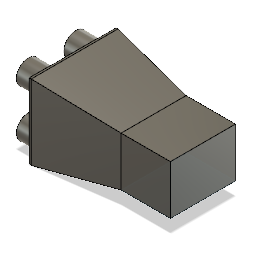
ExtrusionRack_mount_hanging_version (Autodesk Fusion 360 design; units mm, degrees)
Autodesk Fusion 360 part; units mm, degrees
sketch "Sketch1" plane through (0, 0, 0) normal (0, 0, 1) x (1, 0, 0)
  line L0 (10.25, -10.25) -> (-10.25, -10.25)
  line L1 (-10.25, -10.25) -> (-10.25, 10.25)
  line L2 (-10.25, 10.25) -> (10.25, 10.25)
  line L3 (10.25, 10.25) -> (10.25, -10.25)
  line L4 (10.25, -10.25) -> (-10.25, 10.25) construction
  line L5 (-10.25, -10.25) -> (10.25, 10.25) construction
  line L6 (12.5, -12.5) -> (-12.5, -12.5)
  line L7 (-12.5, -12.5) -> (-12.5, 12.5)
  line L8 (-12.5, 12.5) -> (12.5, 12.5)
  line L9 (12.5, 12.5) -> (12.5, -12.5)
  line L10 (12.5, -12.5) -> (-12.5, 12.5) construction
  line L11 (-12.5, -12.5) -> (12.5, 12.5) construction
  dimension "d1" = 20.5
  dimension "d2" = 20.5
  dimension "d3" = 25
  dimension "d4" = 25
  constraint perpendicular L0 L1
  constraint parallel L0 L2
  constraint parallel L1 L3
  constraint horizontal L0
  constraint coincident L4 origin
  constraint coincident L5 origin
  constraint perpendicular L6 L7
  constraint parallel L6 L8
  constraint parallel L7 L9
  constraint horizontal L6
  constraint coincident L10 origin
  constraint coincident L11 origin
  measures "d1" distance of L1.end L2.end
  measures "d2" distance of L0.end L1.end
  measures "d3" distance of L7.end L8.end
  measures "d4" distance of L6.end L7.end
extrude "Extrude1" add sketch "Sketch1" along normal blind 30 makes body 1
sketch "Sketch2" plane through (0, 0, 30) normal (0, 0, 1) x (1, 0, 0)
  line L0 (-10.25, 10.25) -> (10.25, 10.25)
  line L1 (10.25, 10.25) -> (10.25, -10.25)
  line L2 (10.25, -10.25) -> (-10.25, -10.25)
  line L3 (-10.25, -10.25) -> (-10.25, 10.25)
  line L4 (12.5, 12.5) -> (-12.5, 12.5)
  line L5 (-12.5, 12.5) -> (-12.5, -12.5)
  line L6 (-12.5, -12.5) -> (12.5, -12.5)
  line L7 (12.5, -12.5) -> (12.5, 12.5)
  line L8 (-12.5, 12.5) -> (12.5, 12.5)
  line L9 (12.5, 12.5) -> (12.5, -12.5)
  line L10 (12.5, -12.5) -> (-12.5, -12.5)
  line L11 (-12.5, -12.5) -> (-12.5, 12.5)
  constraint horizontal L8
  constraint vertical L9
  constraint horizontal L10
  constraint vertical L11
  constraint coincident L6.end L7.start
  constraint coincident L4.end L5.start
extrude "Extrude2" add sketch "Sketch2" along normal blind 3 contours L0 L1 L2 L3 | L4 L5 L6 L7 L8 L9 L10 L11 bodies 1
sketch "Sketch7" plane through (0, -12.5, 0) normal (0, -1, 0) x (1, 0, 0)
  line L0 (-12.5, 0) -> (12.5, 0)
  line L1 (12.5, 0) -> (12.5, 33)
  line L2 (12.5, 33) -> (-12.5, 33)
  line L3 (-12.5, 33) -> (-12.5, 0)
ref_plane "WorkPlane3" through (0, -0.5, 16.5) normal (0, -1, 0) x (1, 0, 0)
sketch "Sketch8" plane through (0, -0.5, 16.5) normal (0, -1, 0) x (1, 0, 0)
ref_plane "WorkPlane4" through (-52.5, 0, 16.5) normal (-1, 0, 0) x (0, -1, 0)
sketch "Sketch9" plane through (-52.5, 0, 16.5) normal (-1, 0, 0) x (0, 0, -1)
  line L0 (-22, 19) -> (22, 19)
  line L1 (22, 19) -> (22, -19)
  line L2 (22, -19) -> (-22, -19)
  line L3 (-22, -19) -> (-22, 19)
  line L4 (-22, 19) -> (22, -19) construction
  line L5 (22, 19) -> (-22, -19) construction
  constraint perpendicular L0 L1
  constraint parallel L0 L2
  constraint parallel L1 L3
  constraint horizontal L0
  constraint coincident L4 origin
  constraint coincident L5 origin
extrude "Extrude4" add sketch "Sketch9" along normal blind 1 separate body makes body 2
loft "Loft2" add section 1 face at (-12.5, -4.1667, 11) section 2 face at (-52.5, -6.3333, 23.8333) on bodies 1 2 bodies 1 2
sketch "Sketch10" plane through (-53.5, 0, 0) normal (-1, 0, 0) x (0, 0, 1)
  line L0 (38.5, 19) -> (-5.5, 19)
  line L1 (-5.5, 19) -> (-5.5, -19)
  line L2 (-5.5, -19) -> (38.5, -19)
  line L3 (38.5, -19) -> (38.5, 19)
  circle A0 centre (5, 12) radius 6.05
  circle A1 centre (29.05, 12) radius 6.05
  circle A2 centre (5, -12.05) radius 6.05
  circle A3 centre (29.05, -12.05) radius 6.05
  dimension "d18" = 12.1
  dimension "d21" = 24.05
  dimension "d22" = -24.05
  measures "d18" diameter of A0
extrude "Extrude5" add sketch "Sketch10" along normal blind 10 contours A0 | A1 | A2 | A3 bodies 1
equation "d21 = 17.75 mm + ( ( 12.6 / 2 ) * 1 mm )"
equation "d22 = -( 17.75 mm + ( ( 12.6 / 2 ) * 1 mm ) )"
